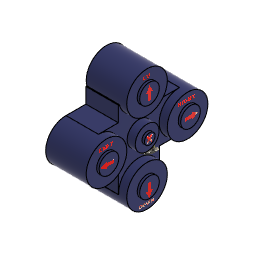
Grup4_Lab4_Palanca_Pruebas v2 (Autodesk Fusion 360 design; units mm, degrees)
Autodesk Fusion 360 part; units mm, degrees
sketch "Boceto1" plane through (0, 0, 0) normal (1, 0, 0) x (0, 1, 0)
  circle A0 centre (0, 25) radius 25
  circle A1 centre (50, -25) radius 25
  circle A2 centre (-50, -25) radius 25
  circle A3 centre (0, -75) radius 25
  line L0 (-50, 0) -> (-25, 0)
  line L1 (-25, 0) -> (-25, 20)
  line L2 (24.4949, 0) -> (50, 0)
  line L3 (24.4949, 0) -> (24.4949, 20)
  line L4 (-50, -50) -> (-25, -50)
  line L5 (-25, -50) -> (-25, -75)
  line L6 (25, -75) -> (25, -50)
  line L7 (25, -50) -> (50, -50)
  circle A4 centre (0.159, -23.7055) radius 14.6817
  constraint coincident A2 L0.start
  constraint tangent A2 L0
  constraint horizontal L0
  constraint perpendicular L0 L1
  constraint coincident A0 L3.end
  constraint coincident A1 L2.end
  constraint tangent A1 L2
  constraint coincident A2 L4.start
  constraint tangent A2 L4
  constraint perpendicular L3 L4
  constraint coincident A3 L5.end
  constraint tangent A3 L5
  constraint perpendicular L4 L5
  constraint coincident A3 L6.start
  constraint tangent A3 L6
  constraint perpendicular L4 L6
  constraint coincident A1 L7.end
  constraint tangent A1 L7
  constraint perpendicular L6 L7
extrude "Extruir1" add sketch "Boceto1" along normal blind 50 makes body 1 at (16.6667, 74.8758, -27.4892) makes body 2 at (16.6667, -25.1242, -27.4892) makes body 3 at (16.6667, 14.7677, -25.1673) makes body 4 at (16.6667, 24.8758, 22.5108) makes body 5 at (16.6667, 24.8758, -77.4892)
sketch "Boceto2" plane through (0, 0, 0) normal (1, 0, 0) x (0, 1, 0)
  line L0 (25.4022, 18.8165) -> (25.0259, 18.8165)
  line L1 (25.0259, -76.7712) -> (25.4022, -76.7712)
  line L2 (25.4022, -76.7712) -> (25.4022, 18.8165)
  line L3 (-25.4022, -76.7712) -> (25.4022, -76.7712)
  line L4 (25.4022, -76.7712) -> (25.4022, 18.8165)
  line L5 (25.4022, 18.8165) -> (-25.4022, 18.8165)
  line L6 (-25.4022, 18.8165) -> (-25.4022, -76.7712)
  line L7 (50, 0) -> (-50, 0)
  line L8 (-50, 0) -> (-50, -50)
  line L9 (-50, -50) -> (50, -50)
  line L10 (50, -50) -> (50, 0)
  constraint horizontal L0
  constraint horizontal L1
  constraint vertical L2
  constraint horizontal L3
  constraint vertical L4
  constraint horizontal L5
  constraint vertical L6
  constraint horizontal L7
  constraint vertical L8
  constraint horizontal L9
  constraint vertical L10
extrude "Extruir2" cut sketch "Boceto2" along normal blind 40 contours L2 L4 L7 L9 L10 bodies 1
extrude "Extruir3" add sketch "Boceto2" along normal blind 40 contours L2 L4 L7 L9 L10 bodies 1
extrude "Extruir4" cut sketch "Boceto2" along normal blind 40 contours L0 L2 L4 L5 L6 L7 bodies 4
extrude "Extruir5" add sketch "Boceto2" along normal blind 40 contours L0 L2 L4 L5 L6 L7 bodies 4
extrude "Extruir6" cut sketch "Boceto2" along normal blind 40 contours L1 L2 L3 L4 L6 L9 bodies 5
extrude "Extruir7" add sketch "Boceto2" along normal blind 40 contours L1 L2 L3 L4 L6 L9 bodies 5
extrude "Extruir8" cut sketch "Boceto2" along normal blind 40 contours L6 L7 L8 L9 bodies 2
extrude "Extruir9" add sketch "Boceto2" along normal blind 40 contours L6 L7 L8 L9 bodies 2 4 5
extrude "Extruir10" cut sketch "Boceto2" along normal blind 40 contours L2 L4 L6 L7 L9 bodies 1 2 3
extrude "Extruir11" add sketch "Boceto2" along normal blind 40 contours L2 L4 L6 L7 L9 bodies 1 2 3
sketch "Boceto3" plane through (0, 0, 0) normal (1, 0, 0) x (0, 1, 0)
sketch "Boceto8" plane through (50, 0, 0) normal (1, 0, 0) x (0, 1, 0)
  circle A0 centre (0, 25) radius 25
  circle A1 centre (0, 25) radius 12.084
  circle A2 centre (50.6241, -25.0998) radius 12.084
  circle A3 centre (0.316, -23.4452) radius 6.5624
  circle A4 centre (0, 25) radius 12.084
  circle A5 centre (-50, -25) radius 12.084
  circle A6 centre (0, -75) radius 12.084
  dimension "d31" = 24.168
  dimension "d48" = 24.168
  dimension "d49" = 24.168
  measures "d31" diameter of A2
  measures "d48" diameter of A5
  measures "d49" diameter of A6
extrude "Extruir12" add sketch "Boceto8" along normal blind 20 contours A1 A4 bodies 1
delete_face "SuprimirCaras2" 1 faces at (63.3333, 12.069, 24.3977) on bodies 1
extrude "Extruir13" add sketch "Boceto8" along normal blind 3 contours A1 A4 bodies 1
extrude "Extruir14" add sketch "Boceto8" along normal blind 3 contours A3 bodies 1
extrude "Extruir15" add sketch "Boceto8" along normal blind 3 contours A2 bodies 1
sketch "Boceto10" plane through (0, 0, 0) normal (1, 0, 0) x (0, 1, 0)
extrude "Extruir16" add sketch "Boceto8" along normal blind 3 contours A5 bodies 1
extrude "Extruir17" add sketch "Boceto8" along normal blind 3 contours A6 bodies 1
copy_body "Cuerpo - > Comp.1" bodies 1 removing the originals makes body 6 in component "Component"
sketch "Boceto11" plane through (0, 0, 0) normal (1, 0, 0) x (0, 1, 0)
sketch "Boceto12" plane through (0, 0, 0) normal (1, 0, 0) x (0, 1, 0)
component "Component" placed x (1, 0, 0) y (0, 1, 0) z (0, 0, 1) at (1.1259, 0.6556, -7.5271)
